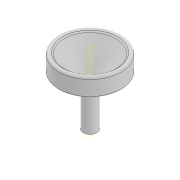
# Autodesk Inventor part: Electrode Funnel v0.6.2
Saved by Autodesk Inventor 2022 (Build 260153000, 153)
## iProperties
Created: 2023-06-02
Part Number: Electrode Funnel v0.6.2
Material: Generic
Document SubType Name: Modeling
Designer: cheap
Density: 1 g/cm^3
Appearance: Default
Author: cheap
Autodesk Inventor part; units mm, degrees
ref_plane "YZ Plane" through (0, 0, 0) normal (1, 0, 0) x (0, 1, 0)
ref_plane "XZ Plane" through (0, 0, 0) normal (0, 1, 0) x (-1, 0, 0)
ref_plane "XY Plane" through (0, 0, 0) normal (0, 0, 1) x (1, 0, 0)
sketch "Sketch1" plane through (0, 0, 0) normal (0, 0, 1) x (1, 0, 0)
  line L0 (0, 0) -> (4.44, 0)
  line L1 (4.44, 0) -> (4.44, 44)
  line L2 (4.44, 44) -> (-0.05, 44)
  line L3 (-0.05, 44) -> (-2.0503, 34.9996)
  line L4 (-0.05, 44) -> (9.17, 44) construction
  line L5 (-2.0503, 34.9996) -> (-2.0503, 30.0996) construction
  arc A0 (-2.0503, 34.9996) -> (-2.0503, 30.0996) centre (6.4601, 32.5496) ccw
  line L6 (-2.0503, 30.0996) -> (-0.0024, 35.1178)
  line L7 (-2.0503, 30.0996) -> (3.3697, 30.0996) construction
  line L8 (-0.0024, 35.1178) -> (0, 0)
  line L9 (0, 0) -> (4.44, 0)
  line L10 (-3.0503, 44) -> (-3.0503, 0) construction
  dimension "d0" = 4.44
  dimension "d1" = 44
  dimension "d2" = 4.49
  dimension "d5" = 9.22
  dimension "d6" = 102.53
  dimension "d7" = 4.9
  dimension "d8" = 5.42
  dimension "d9" = 67.8
  dimension "d10" = 1
  constraints: 22 end point, 4 horizontal, 2 equal length, 2 point on circle, 2 vertical, 1 centre point, 1 perpendicular
  measures "d0" distance of L0.start L0.end
  measures "d1" distance of L0.end L1.end
  measures "d2" distance of L1.end L2.end
  measures "d5" distance of L2.end L3.end
  measures "d6" angle of L3 L4
  measures "d7" distance of L3.end L5.end
  measures "d8" distance of L5.end L6.end
  measures "d9" angle of L7 L6
  measures "d10" distance from line of L10 L5.end
revolve "Revolution1" add sketch "Sketch1" angle 360 about axis through (-3.0503, 44, 0) along (0, -1, 0)
sketch "Sketch2" plane through (0, 0, 0) normal (0, 0, 1) x (1, 0, 0)
  line L0 (-2.0503, 34.9996) -> (-0.05, 44) projected
  arc A0 (31.5525, 72.1787) -> (27.3386, 73.803) centre (29.1325, 72.1787) ccw
  line L1 (25.8474, 72.6089) -> (27.3386, 73.803)
  line L2 (31.5525, 72.1787) -> (31.5525, 55.7587)
  line L3 (30.5525, 54.7587) -> (28.1425, 54.7587)
  line L4 (27.1425, 55.7587) -> (27.1425, 59.7587)
  line L5 (27.1425, 59.7587) -> (21.8425, 59.7587)
  line L6 (21.8425, 59.7587) -> (21.8425, 55.1732)
  line L7 (4.44, 37.37) -> (21.5493, 54.4658)
  arc A1 (27.1425, 55.7587) -> (28.1425, 54.7587) centre (28.1425, 55.7587) ccw
  arc A2 (30.5525, 54.7587) -> (31.5525, 55.7587) centre (30.5525, 55.7587) ccw
  line L8 (-6.0506, 44) -> (-0.05, 44) projected
  line L9 (-0.05, 44) -> (4.44, 44)
  arc A3 (21.5493, 54.4658) -> (21.8425, 55.1732) centre (20.8425, 55.1732) ccw
  line L10 (-0.05, 44) -> (4.44, 44)
  line L11 (4.44, 44) -> (4.44, 37.37)
  line L12 (4.44, 44) -> (4.44, 0) projected
  line L13 (25.8474, 72.6089) -> (-0.05, 44)
  line L14 (-3.0503, -1.6042) -> (-3.0503, 46.7159) construction
  point P0 (0, 0)
  point P1 (31.5525, 54.7587)
  point P2 (27.1425, 54.7587)
  dimension "d14" = 4.84
  dimension "d16" = 17.42
  dimension "d18" = 4.41
  dimension "d19" = 5
  dimension "d20" = 5.3
  dimension "d21" = 6.63
  dimension "d22" = 1
  dimension "d23" = 1
  constraints: 24 end point, 8 point on circle, 7 tangent, 4 centre point, 4 point on line, 3 horizontal, 2 perpendicular, 2 vertical, 1 collinear, 1 equal radius
  measures "d14" diameter of A0
  measures "d16" distance of L2.start point (31.552, 54.759)
  measures "d18" distance of point (31.552, 54.759) point (27.142, 54.759)
  measures "d19" distance of point (27.142, 54.759) L4.end
  measures "d20" distance of L4.end L5.end
  measures "d21" distance of L11.start L7.start
  measures "d22" radius of A1
  measures "d23" radius of A3
revolve "Revolution2" add sketch "Sketch2" angle 360 about axis through (-3.0503, -1.6042, 0) along (0, 1, 0)
body "Solid1"
